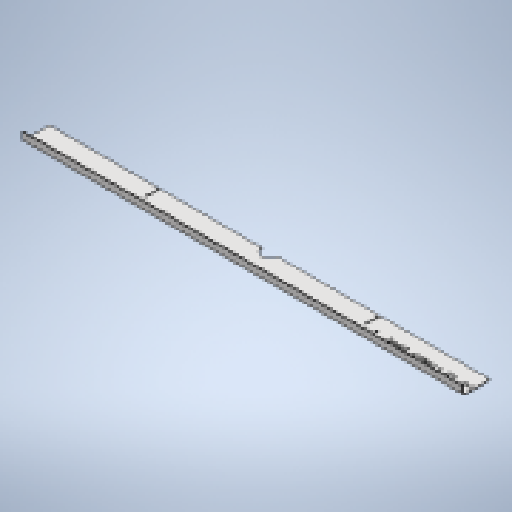
# Autodesk Inventor part: MSC 341 stringer BOARD  #
Saved by Autodesk Inventor 2025.1 (Build 291241020, 241B)
## iProperties
Created: 2024-04-28
Part Number: MSC 341 stringer BOARD  #
Material: Stainless Steel
Document SubType Name: Sheet Metal
Designer: admin
Stock Number: МОО 341 стрингер борт #
Density: 8 g/cm^3
Flat Pattern Width: 98 cm
Flat Pattern Length: 7.7202 cm
Flat Pattern Area: 756.58 cm^2
Sheet Metal Rule: AISI304 2mm Die16
Sheet Metal Width: 980.000 mm
Sheet Metal Length: 77.202 mm
Sheet Metal Area: 75657.951 mm^2
Appearance: Default
Mass: 1196.16 g
Surface Area: 1540.97 cm^2
Volume: 149.52 cm^3
Description: DIE16(5)|\ 90°|corrY -___°|X_____|bom___
Author: admin
Autodesk Inventor part; units mm, degrees
ref_plane "YZ Plane" through (0, 0, 0) normal (1, 0, 0) x (0, 1, 0)
ref_plane "XZ Plane" through (0, 0, 0) normal (0, 1, 0) x (-1, 0, 0)
ref_plane "XY Plane" through (0, 0, 0) normal (0, 0, 1) x (1, 0, 0)
sketch "Sketch1" plane through (0, 0, 0) normal (0, 0, 1) x (1, 0, 0)
  line L0 (-490, 59) -> (490, 59)
  line L1 (490, 59) -> (490, 0)
  line L2 (490, 0) -> (-490, 0)
  line L3 (-490, 0) -> (-490, 59)
  point P0 (0, 0)
  point P1 (0, 0)
  dimension "d0" = 980
  dimension "d1" = 59
  measures "d0" distance of L1.end L2.end
  measures "d1" distance of L0.end L1.end
extrude "Plate1" add sketch "Sketch1" along normal blind 2
sketch "Sketch2" plane through (490, -2, 0) normal (0, 1, 0) x (-1, 0, 0)
  line L0 (980, 0) -> (0, 0)
  line L1 (0, 0) -> (0, 20)
  line L2 (0, 20) -> (980, 20)
  line L3 (980, 20) -> (980, 0)
  constraints: 6 end point, 1 horizontal, 1 perpendicular, 1 vertical
edge flange "Flange1" height 20 angle 90 thickness 2 bend radius 2.75 thickness toward (0, 1, 0) relief round relief width 2 relief depth 1 edges at (0, 0, 2) wall of the first edge with corners at (-490, -2, 0) (490, -2, 0) (490, -2, 20) (-490, -2, 20)
bend "Bend1"
corner "Corner1"
sketch "Sketch5" plane through (0, 0, 0) normal (0, 0, -1) x (-1, 0, 0)
  line L0 (490, 59) -> (-490, 59) projected
  line L1 (490, -2) -> (-490, -2) projected
  circle A0 centre (0, 59) radius 17.5
  line L2 (243.4, 59) -> (246.6, 59)
  line L3 (246.6, 59) -> (246.6, 26)
  line L4 (246.6, 26) -> (243.4, 26)
  line L5 (243.4, 26) -> (243.4, 59)
  line L6 (-243.4, 59) -> (-246.6, 59)
  line L7 (-246.6, 59) -> (-246.6, 26)
  line L8 (-246.6, 26) -> (-243.4, 26)
  line L9 (-243.4, 26) -> (-243.4, 59)
  line L10 (0, 59) -> (0, -2) construction
  point P0 (0, 0)
  point P1 (-490, -2)
  point P2 (245, 26)
  point P3 (-245, 26)
  point P4 (246.6, 59)
  point P5 (-17.5, 59)
  point P6 (17.5, 59)
  point P7 (-246.6, 59)
  dimension "d45" = 35
  dimension "d48" = 3.2
  dimension "d49" = 490
  dimension "d51" = 28
  dimension "d52" = 33
  constraints: 18 end point, 4 parallel, 3 midpoint, 2 collinear, 2 horizontal, 2 perpendicular, 2 point on line, 1 centre point, 1 vertical, 3 other
  measures "d45" diameter of A0
  measures "d48" distance of L7.end L8.end
  measures "d49" distance of point (245, 26) point (-245, 26)
  measures "d52" distance between parallel lines of L0 L8
extrude "Extrusion1" cut sketch "Sketch5" against normal through all contours L3 L4 L5 L0 | L9 L8 L7 L0 | A0 L0 picked at (-2.238, 52.1497)
sketch "Sketch9" plane through (0, 0, 2) normal (0, 0, 1) x (1, 0, 0)
  line L0 (485.6141, 29.596) -> (485.6141, 17.596) construction
  line L1 (485.6141, 17.596) -> (285.6141, 17.596) construction
  line L2 (285.6141, 17.596) -> (285.6141, 29.596) construction
  line L3 (285.6141, 29.596) -> (485.6141, 29.596) construction
  line L4 (-490, 59) -> (490, 59) projected
  point P0 (0, 0)
  point P1 (1.05, 68)
  point P2 (490, 59)
  dimension "d40" = 200
  dimension "d41" = 12
  constraints: 1 horizontal, 3 other
  measures "d40" distance of L0.end L1.end
  measures "d41" distance of L1.end L2.end
mark "Mark2"
equation "\"d2\" = Thickness"
equation "\"d3\" = BendReliefWidth"
equation "\"d4\" = BendReliefDepth"
equation "\"d5\" = MinimumRemnant"
equation "\"d6\" = TransitionRadius"
equation "\"d9\" = BendRadius"
equation "\"d10\" = CornerReliefSize"
equation "\"d11\" = GapSize"
equation "\"d12\" = JacobiRadiusSize"
equation "\"BendReliefWidth\" = Thickness"
equation "\"BendReliefDepth\" = 0.5 * Thickness"
equation "\"CornerReliefSize\" = 4 * Thickness"
equation "\"MinimumRemnant\" = 2 * Thickness"
equation "\"TransitionRadius\" = BendRadius"
equation "\"JacobiRadiusSize\" = BendRadius"
equation "\"GapSize\" = Thickness"
equation "\"Thickness\" = 2"
equation "\"BendRadius\" = 2.75"
body "Solid1"
